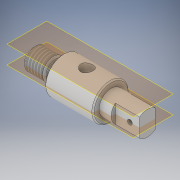
# Autodesk Inventor part: вал
Saved by Autodesk Inventor 2019.4 (Build 234330000, 330)
## iProperties
Created: 2020-05-06
Part Number: вал
Material: Типовые
Document SubType Name: Modeling
Designer: Asus
Density: 1 g/cm^3
Appearance: По умолчанию
Mass: 40.3359 g
Surface Area: 88.2222 cm^2
Volume: 40.3359 cm^3
Author: Asus
Autodesk Inventor part; units mm, degrees
ref_plane "YZ Plane" through (0, 0, 0) normal (1, 0, 0) x (0, 1, 0)
ref_plane "XY Plane" through (0, 0, 0) normal (0, 0, 1) x (1, 0, 0)
sketch "Эскиз2" plane through (0, 0, 0) normal (0, 0, 1) x (1, 0, 0)
  line L0 (-45, 0) -> (-45, 9)
  line L1 (-27.75, 9) -> (-45, 9)
  line L2 (-26, 7.25) -> (-20, 7.25)
  line L3 (-20, 7.25) -> (-20, 14)
  line L4 (-19, 15) -> (20, 15)
  line L5 (-26, 7.25) -> (-27.75, 9)
  line L6 (50, 10) -> (50, 0)
  line L7 (50, 10) -> (20, 10)
  line L8 (20, 10) -> (20, 14)
  line L9 (-45, 0) -> (50, 0)
  line L10 (-20, 14) -> (-20, 15)
  line L11 (-20, 15) -> (-19, 15)
  line L12 (20, 15) -> (20, 14)
  point P0 (0, 0)
  point P1 (0, 15)
  dimension "d1" = 9
  dimension "d15" = 6
  dimension "d16" = 19
  dimension "d22" = 10
  dimension "d23" = 20
  dimension "d41" = 25
  dimension "d42" = 17.25
  dimension "d57" = 20
  dimension "d58" = 70
  constraints: 26 end point, 4 horizontal, 3 vertical, 2 perpendicular, 1 collinear, 1 point on line
  measures "d1" distance of L0.start L0.end
  measures "d15" distance of L2.end L2.start
  measures "d16" horizontal distance of L0.end L2.start
  measures "d22" distance of L6.start L6.end
  measures "d23" horizontal distance of L3.end point (0, 15)
  measures "d41" horizontal distance of L2.end L0.start
  measures "d42" distance of L1.start L0.end
  measures "d57" distance from line of point (0, 15) L12
  measures "d58" distance between parallel lines of L6 L3
revolve "Вращение1" add sketch "Эскиз2" angle 360 about axis through (-45, 0, 0) along (1, 0, 0)
sketch "Эскиз3" plane through (0, 0, 0) normal (0, 1, 0) x (-1, 0, 0)
  line L0 (-50, -10) -> (-30, -10)
  line L1 (-30, -10) -> (-30, -6.5)
  line L2 (-30, -6.5) -> (-50, -6.5)
  line L3 (-50, -6.5) -> (-50, -10)
  line L4 (-50, 10) -> (-30, 10)
  line L5 (-30, 10) -> (-30, 6.5)
  line L6 (-30, 6.5) -> (-50, 6.5)
  line L7 (-50, 6.5) -> (-50, 10)
  point P0 (0, 0)
  constraints: 16 end point, 4 parallel, 2 horizontal, 2 perpendicular
extrude "Выдавливание1" cut sketch "Эскиз3" along normal mid plane 44.25
sketch "Эскиз4" plane through (0, 0, 0) normal (0, 0, 1) x (1, 0, 0)
  line L0 (50, 7.5993) -> (50, -7.5993) projected
  point P0 (0, 0)
  point P1 (42, 0)
hole "Отверстие1" at (42, 0, 0) direction (0, 0, -1) diameter 4 end through all both
thread "Резьба1" size "M18x2.5" class "6g" standard "ISO Metric profile" full length
chamfer "Фаска1" distance 2.5 angle 45 1 edges at (-45, -9, 0)
ref_plane "РабПлоскость1" through (0, 15, 0) normal (0, 1, 0) x (-1, 0, 0)
fillet "Сопряжение1" radius 1.6 1 edges at (-20, -7.25, 0)
fillet "Сопряжение2" radius 1 1 edges at (-26, -7.25, 0)
chamfer "Фаска2" distance 1 angle 45 2 edges at (20, -15, 0) (-20, -15, 0)
sketch "Эскиз6" plane through (0, 15, 0) normal (0, 1, 0) x (-1, 0, 0)
  point P0 (0, 0)
  point P1 (0, 0)
  constraints: 1 coincident
hole "Отверстие3" at (0, 15, 0) direction (0, -1, 0) diameter 10 depth 15 tip angle 118
